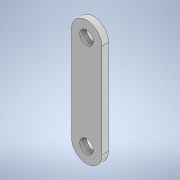
# Autodesk Inventor part: zawieszenie ramie
Saved by Autodesk Inventor 2021 (Build 250183000, 183)
## iProperties
Created: 2021-06-24
Part Number: zawieszenie ramie
Material: Generic
Document SubType Name: Modeling
Designer: Łukasz
Density: 1 g/cm^3
Appearance: Default
Author: Łukasz
Autodesk Inventor part; units mm, degrees
ref_plane "YZ Plane" through (0, 0, 0) normal (1, 0, 0) x (0, 1, 0)
ref_plane "XZ Plane" through (0, 0, 0) normal (0, 1, 0) x (-1, 0, 0)
ref_plane "Work Plane1" through (0, 0, 3.5) normal (0, 0, 1) x (1, 0, 0)
sketch "Sketch2" plane through (0, 0, 3.5) normal (0, 0, 1) x (1, 0, 0)
  circle A0 centre (0, 0) radius 13 projected
  line L0 (13, 0) -> (-13, 0)
  line L1 (-13, 0) -> (-13, 65)
  line L2 (-13, 65) -> (13, 65)
  line L3 (13, 65) -> (13, 0)
  line L4 (9, 0) -> (-9, 0)
  line L5 (-9, 0) -> (-9, 65)
  line L6 (-9, 65) -> (9, 65)
  line L7 (9, 65) -> (9, 0)
  point P0 (9, 9.3808)
  point P1 (9, 65)
  point P2 (-9, 9.3808)
  dimension "d5" = 65
  dimension "d15" = 18
  constraints: 16 end point, 4 parallel, 2 horizontal, 2 perpendicular, 2 point on line, 2 other
  measures "d5" distance of L0.end L1.end
  measures "d15" distance of L5.end L6.end
extrude "Extrusion2" add sketch "Sketch2" along normal blind 2 and the other way blind 2 contours L5 L2 L7 A0
fillet "Fillet1" radius 9 2 edges at (9, 65, 3.5) (-9, 65, 3.5)
sketch "Sketch3" plane through (0, 0, 5.5) normal (0, 0, 1) x (1, 0, 0)
  circle A0 centre (0, 56) radius 4
  arc A1 (9, 56) -> (-9, 56) centre (0, 56) ccw projected
  point P0 (0, 0)
  dimension "d11" = 8
  dimension "d17" = 0
  constraints: 1 centre point
  measures "d11" diameter of A0
  measures "d17" distance of A1.centre A0.centre
extrude "Extrusion3" cut sketch "Sketch3" against normal up to surface (4 mm away)
sketch "Sketch4" plane through (0, 0, 5.5) normal (0, 0, 1) x (1, 0, 0)
  circle A0 centre (0, 0) radius 11 projected
  circle A1 centre (0, 0) radius 4
  circle A2 centre (0, 0) radius 9
  line L0 (9, 9.3808) -> (9, 56) projected
  line L1 (9, 0) -> (9, 9.3808)
  line L2 (-9, 0) -> (-9, 9.8723)
  line L3 (-9, 56) -> (-9, 9.3808) projected
  line L4 (9, 9.3808) -> (4, 16.3545)
  line L5 (4, 16.3545) -> (-2.5597, 14.9818)
  line L6 (-2.5597, 14.9818) -> (-9, 9.8723)
  dimension "d18" = 8
  dimension "d19" = 18
  constraints: 10 end point, 2 centre point, 2 coincident, 2 point on circle, 1 collinear, 1 point on line
  measures "d18" diameter of A1
  measures "d19" diameter of A2
extrude "Extrusion4" add sketch "Sketch4" against normal blind 4 contours L1 A2 L2 A0 | A0 L2 L6 L5 L4 L1 | A2 picked at (7.6596, 6.8574)
body "Solid1"
